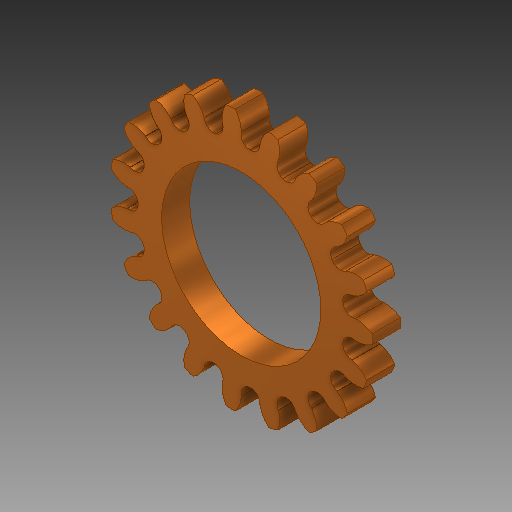
# Autodesk Inventor part: UltrasonicGear
Saved by Autodesk Inventor 2017 (Build 210142000, 142)
## iProperties
Created: 2017-02-15
Part Number: UltrasonicGear
Material: Gold
Document SubType Name: Modeling
Designer: Moonlight.Admin
Density: 19.3 g/cm^3
Appearance: Metal 1600F Hot
Author: Moonlight.Admin
Autodesk Inventor part; units mm, degrees
ref_plane "YZ Plane" through (0, 0, 0) normal (1, 0, 0) x (0, 1, 0)
ref_plane "XZ Plane" through (0, 0, 0) normal (0, 1, 0) x (-1, 0, 0)
ref_plane "XY Plane" through (0, 0, 0) normal (0, 0, 1) x (1, 0, 0)
derived "CombinedHousingV2.ipt"
sketch "UltrasonicBase" plane through (0, 0, 0) normal (0, 0, 1) x (1, 0, 0)
  line L0 (-10.8, -29.125) -> (36.2, -29.125)
  line L1 (36.2, -29.125) -> (36.2, -50.625)
  line L2 (36.2, -50.625) -> (-10.8, -50.625)
  line L3 (-10.8, -50.625) -> (-10.8, -29.125)
  line L4 (-25.125, -25.125) -> (-25.125, 25.125) construction
  line L5 (25.125, -25.125) -> (-25.125, -25.125) construction
  circle A0 centre (-0.3, -39.875) radius 8.5
  circle A1 centre (25.7, -39.875) radius 8.5
  line L6 (12.7, -50.625) -> (12.7, -29.125) construction
  line L7 (6.35, -50.625) -> (6.35, -45.625)
  line L8 (6.35, -45.625) -> (19.05, -45.625)
  line L9 (19.05, -45.625) -> (19.05, -50.625)
  arc A2 (8.95, -30.125) -> (8.95, -36.125) centre (8.95, -33.125) ccw
  arc A3 (16.45, -36.125) -> (16.45, -30.125) centre (16.45, -33.125) ccw
  line L10 (8.95, -36.125) -> (16.45, -36.125)
  line L11 (8.95, -30.125) -> (16.45, -30.125)
  arc A4 (8.95, -36.125) -> (8.95, -30.125) centre (8.95, -33.125) ccw construction
  arc A5 (16.45, -30.125) -> (16.45, -36.125) centre (16.45, -33.125) ccw construction
  circle A6 centre (-17.3, -39.875) radius 1.905
  circle A7 centre (-17.3, -39.875) radius 5
  circle A8 centre (42.7, -39.875) radius 1.905
  circle A9 centre (42.7, -39.875) radius 5
  point P0 (0, 0)
  point P1 (12.7, -39.875)
sketch "Sketch2" plane through (0, 0, 0) normal (0, 0, 1) x (1, 0, 0)
  arc A0 (39.6726, -40.375) -> (39.6726, -39.375) centre (36.7145, -39.875) ccw
  line L0 (39.6726, -40.375) -> (39.6726, -39.375) construction
  line L1 (37.6726, -40.875) -> (37.6726, -38.875) construction
  line L2 (40.1726, -42.8653) -> (40.1726, -36.8847)
  arc A1 (37.6726, -40.875) -> (39.6726, -40.375) centre (38.0542, -38.1516) ccw
  line L3 (37.5338, -42.8653) -> (40.1726, -42.8653)
  line L4 (40.1726, -36.8847) -> (37.5338, -36.8847)
  arc A2 (37.6726, -40.875) -> (37.5338, -42.8653) centre (37.5338, -41.8653) ccw
  arc A3 (37.5338, -36.8847) -> (37.6726, -38.875) centre (37.5338, -37.8847) ccw
  arc A4 (39.6726, -39.375) -> (37.6726, -38.875) centre (38.0542, -41.5984) ccw
  circle A5 centre (25.7, -39.875) radius 11 construction
  circle A6 centre (25.7, -39.875) radius 14.0145
  line L5 (25.4766, -39.875) -> (31.7358, -39.875) construction
  circle A7 centre (25.7, -39.875) radius 8.5 projected
  circle A8 centre (-0.3, -39.875) radius 8.5 projected
  circle A9 centre (-0.3, -39.875) radius 11 construction
  point P0 (0, 0)
  point P1 (37.6726, -39.875)
  point P2 (39.6726, -39.875)
  dimension "d1" = 3
  dimension "d2" = 2
  dimension "d3" = 0.5
  dimension "d4" = 1
  dimension "d5" = 2
  dimension "d6" = 2.75
  dimension "d7" = 1
  dimension "d9" = 22
  constraints: 13 end point, 10 point on circle, 8 centre point, 6 tangent, 3 coincident, 3 equal radius, 3 point on line, 2 midpoint, 2 parallel, 1 horizontal
  measures "d1" radius of A0
  measures "d2" distance of L1.end L1.start
  measures "d3" distance between parallel lines of L2 L0
  measures "d4" radius of A2
  measures "d5" distance between parallel lines of L0 L1
  measures "d6" radius of A1
  measures "d7" distance of L0.end L0.start
  measures "d9" diameter of A5
extrude "Extrusion1" add sketch "Sketch2" along normal blind 3 contours A1 A2 L3 A6 L4 A3 A4 A0 | A0 A6 L3 A2 A1 | A0 A4 A3 L4 A6
extrude "Extrusion2" cut sketch "Sketch2" along normal blind 7.62 contours A0 A6 L3 A2 A1 | A0 A4 A3 L4 A6 | A6 L4 L2 L3
pattern_circular "Circular Pattern1" count 19 over 360 about axis through (25.7, -39.875, 0) along (0, 0, 1) of "Extrusion2"
body "Solid1"
